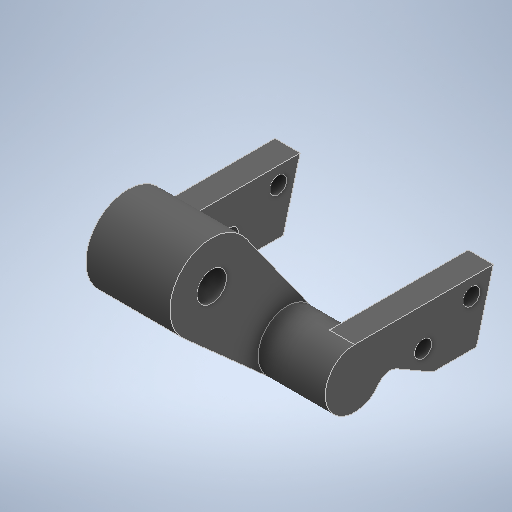
# Autodesk Inventor part: board_setter_joint
Saved by Autodesk Inventor 2026.1 (Build 301233020, 233B)
## iProperties
Created: 2024-10-10
Part Number: board_setter_joint
Material: 一般
Document SubType Name: モデリング
Designer: hibik
Density: 1 g/cm^3
Appearance: 既定
Author: hibik
Autodesk Inventor part; units mm, degrees
ref_plane "YZ Plane" through (0, 0, 0) normal (1, 0, 0) x (0, 1, 0)
ref_plane "XZ Plane" through (0, 0, 0) normal (0, 1, 0) x (-1, 0, 0)
sketch "スケッチ1" plane through (0, 0, 0) normal (1, 0, 0) x (0, 1, 0)
  line L0 (0, 0) -> (10, 0)
  line L1 (10, 0) -> (10, 15)
  line L2 (10, 15) -> (0, 15)
  line L3 (0, 15) -> (0, 0)
  circle A0 centre (6.5, 20) radius 1.6
  circle A1 centre (6.5, 20) radius 3.5
  line L4 (10, 15) -> (-0.0411, 15)
  dimension "d0" = 10
  dimension "d1" = 15
  dimension "d2" = 3.2
  dimension "d3" = 7
  dimension "d7" = 5
  measures "d0" distance of L2.end L1.end
  measures "d1" distance of L1.end L0.end
  measures "d2" diameter of A0
  measures "d3" diameter of A1
  measures "d7" distance from line of L2 A0.centre
extrude "プレート1" add sketch "スケッチ1" along normal blind 1.5
sketch "スケッチ2" plane through (1.5, 0, 0) normal (1, 0, 0) x (0, 0, -1)
  line L0 (-15, 5) -> (-15, 10) projected
  line L1 (-15, 10) -> (-3.4839, 10) projected
  line L2 (-3.4839, 10) -> (-5.4935, 2.5) projected
  line L3 (-5.4935, 2.5) -> (-10.6699, 2.5) projected
  line L4 (-10.6699, 2.5) -> (-15, 5) projected
  line L5 (-15, 10) -> (0, 10) projected
  line L6 (-15, 0) -> (-15, 10) projected
  line L7 (0, 0) -> (-15, 0) projected
  line L8 (0, 10) -> (0, 0) projected
extrude "切り取り1" cut sketch "スケッチ2" against normal blind 1.5 contours L4 L3 L2 L5 L8 L7 L6
sketch "スケッチ3" plane through (1.5, 0, 0) normal (1, 0, 0) x (0, 0, -1)
  line L0 (-3.4839, 10) -> (-15, 10)
  line L1 (-15, 10) -> (-20, 10)
  circle A0 centre (-20, 6.5) radius 3.5
  line L2 (-10.6699, 2.5) -> (-15, 5)
  arc A1 (-15, 5) -> (-17.1135, 4.5206) centre (-15.7977, 3.6183) ccw
  line L3 (-15, 5) -> (-10.6699, 2.5)
  circle A2 centre (-20, 6.5) radius 3.5
  line L4 (-15, 5) -> (-15, 10)
  point P0 (0, 0)
  dimension "d13" = 1.5
  measures "d13" vertical distance of A0.centre L2.end
sheet face with bend "面2" sketch "スケッチ3" thickness 1.5 toward (-1, 0, 0) bend radius 1.5 contours L4 A1 A0 L1
bend "曲げ1"
sketch "スケッチ4" plane through (1.5, 0, 0) normal (1, 0, 0) x (0, 0, -1)
  circle A0 centre (-6.0903, 8) radius 1
  line L0 (-20, 10) -> (-3.4839, 10) projected
  line L1 (-5.4935, 2.5) -> (-3.4839, 10) projected
  circle A1 centre (-11.8349, 5.4821) radius 1
  line L2 (-15, 5) -> (-10.6699, 2.5) projected
  line L3 (-11.8349, 5.4821) -> (-12.8349, 3.75)
  point P0 (0, 0)
  dimension "d14" = 2
  dimension "d15" = 2
  dimension "d16" = 2
  dimension "d17" = 2
  constraints: 2 centre point, 2 end point, 1 equal radius, 1 midpoint, 1 perpendicular
  measures "d14" diameter of A0
  measures "d15" distance from line of L0 A0.centre
  measures "d16" distance from line of L1 A0.centre
  measures "d17" distance from line of L2 L3.start
extrude "切り取り2" cut sketch "スケッチ4" against normal blind 1.5
sketch "スケッチ5" plane through (1.5, 0, 0) normal (1, 0, 0) x (0, 0, -1)
  circle A0 centre (-20, 6.5) radius 3.5
  arc A1 (-20, 10) -> (-17.1135, 4.5206) centre (-20, 6.5) ccw projected
  point P0 (0, 0)
  constraints: 2 concentric, 1 centre point
extrude "押し出し1" add sketch "スケッチ5" against normal blind 11.5
mirror "ミラー1" about plane through (-10, 6.5, 20) normal (-1, 0, 0)
sketch "スケッチ6" plane through (1.5, 0, 0) normal (1, 0, 0) x (0, 0, -1)
  arc A0 (-15, 5) -> (-17.1135, 4.5206) centre (-15.7977, 3.6183) ccw projected
  line L0 (-15, 5) -> (-10.6699, 2.5) projected
  line L1 (-10.6699, 2.5) -> (-5.4935, 2.5) projected
  line L2 (-5.4935, 2.5) -> (-3.4839, 10) projected
  line L3 (-20, 10) -> (-3.4839, 10) projected
  arc A1 (-20, 10) -> (-17.1135, 4.5206) centre (-20, 6.5) ccw projected
  circle A2 centre (-6.0903, 8) radius 1 projected
  circle A3 centre (-11.8349, 5.4821) radius 1 projected
  point P0 (0, 0)
extrude "押し出し2" add sketch "スケッチ6" along normal blind 1.5
sketch "スケッチ7" plane through (-21.5, 10, 3.4839) normal (-1, 0, 0) x (0, 0, 1)
  arc A0 (13.6296, -5.4794) -> (11.5161, -5) centre (12.3138, -6.3817) ccw projected
  arc A1 (13.6296, -5.4794) -> (16.5161, 0) centre (16.5161, -3.5) ccw projected
  line L0 (16.5161, 0) -> (0, 0) projected
  line L1 (2.0096, -7.5) -> (0, 0) projected
  line L2 (7.186, -7.5) -> (2.0096, -7.5) projected
  line L3 (11.5161, -5) -> (7.186, -7.5) projected
  circle A2 centre (2.6065, -2) radius 1 projected
  circle A3 centre (8.3511, -4.5179) radius 1 projected
  point P0 (-3.4839, -10)
extrude "押し出し3" add sketch "スケッチ7" along normal blind 1.5
ref_plane "作業平面1" through (-10, 10, 3.4839) normal (-1, 0, 0) x (0, 0, 1)
sketch "スケッチ8" plane through (-10, 10, 3.4839) normal (-1, 0, 0) x (0, 0, 1)
  circle A0 centre (25.5161, 6.5) radius 5
  arc A1 (13.6296, -5.4794) -> (16.5161, 0) centre (16.5161, -3.5) ccw projected
  line L0 (18.8404, -6.1168) -> (28.8365, 2.7617)
  line L1 (21.4499, 9.4096) -> (13.6698, -1.4633)
  circle A2 centre (16.5161, -3.5) radius 3.5
  arc A3 (16.5161, 0) -> (13.6296, -5.4794) centre (16.5161, -3.5) ccw projected
  point P0 (-3.4839, -10)
  point P1 (13.6698, -1.4633)
  dimension "d26" = 10
  dimension "d27" = 10
  dimension "d28" = 9
  constraints: 4 end point, 4 point on circle, 4 tangent, 1 centre point, 1 coincident, 3 other
  measures "d26" diameter of A0
  measures "d27" vertical distance of A1.centre A0.centre
  measures "d28" horizontal distance of A1.centre A0.centre
extrude "押し出し4" add sketch "スケッチ8" along normal mid plane 10 contours A0 | A0 L0 A1 A2 L1
sketch "スケッチ9" plane through (-5, 10, 3.4839) normal (1, 0, 0) x (0, 0, -1)
  arc A0 (-21.4499, 9.4096) -> (-28.8365, 2.7617) centre (-25.5161, 6.5) ccw projected
  circle A1 centre (-25.5161, 6.5) radius 1.75
  point P0 (3.4839, -10)
  dimension "d31" = 3.5
  constraints: 1 centre point, 1 coincident
  measures "d31" diameter of A1
extrude "押し出し5" cut sketch "スケッチ9" against normal through all
equation "\"d5\" = Thickness"
equation "\"d17\" = d16"
equation "\"d18\" = Thickness"
equation "\"d4\" = Thickness"
equation "\"d8\" = BendRadius"
equation "\"d9\" = BendReliefWidth"
equation "\"d11\" = MinimumRemnant"
equation "\"d10\" = BendReliefDepth"
equation "\"d12\" = TransitionRadius"
equation "\"BendRadius\" = Thickness"
equation "\"BendReliefWidth\" = Thickness"
equation "\"BendReliefDepth\" = 0.5 * Thickness"
equation "\"CornerReliefSize\" = 4 * Thickness"
equation "\"MinimumRemnant\" = 2 * Thickness"
equation "\"TransitionRadius\" = BendRadius"
equation "\"JacobiRadiusSize\" = BendRadius"
equation "\"GapSize\" = Thickness"
equation "\"Thickness\" = 1.5"
